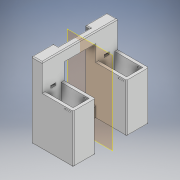
# Autodesk Inventor part: caja_s
Saved by Autodesk Inventor 2020 (Build 240168000, 168)
## iProperties
Created: 2021-01-14
Part Number: caja_s
Material: Generic
Document SubType Name: Modeling
Designer: Gelect
Density: 1 g/cm^3
Appearance: Default
Author: Gelect
Autodesk Inventor part; units mm, degrees
ref_plane "YZ Plane" through (0, 0, 0) normal (1, 0, 0) x (0, 1, 0)
ref_plane "XZ Plane" through (0, 0, 0) normal (0, 1, 0) x (-1, 0, 0)
ref_plane "XY Plane" through (0, 0, 0) normal (0, 0, 1) x (1, 0, 0)
sketch "Sketch1" plane through (0, 0, 0) normal (1, 0, 0) x (0, 1, 0)
  line L0 (38.75, 38.75) -> (-38.75, 38.75)
  line L1 (-38.75, 38.75) -> (-38.75, -38.75)
  line L2 (-38.75, -38.75) -> (38.75, -38.75)
  line L3 (38.75, -38.75) -> (38.75, 38.75)
  line L4 (38.75, 38.75) -> (-38.75, -38.75) construction
  line L5 (-38.75, 38.75) -> (38.75, -38.75) construction
  line L6 (38.75, 16.15) -> (-38.75, 16.15)
  line L7 (-38.75, 16.15) -> (-38.75, -16.15)
  line L8 (-38.75, -16.15) -> (38.75, -16.15)
  line L9 (38.75, -16.15) -> (38.75, 16.15)
  line L10 (38.75, 16.15) -> (-38.75, -16.15) construction
  line L11 (-38.75, 16.15) -> (38.75, -16.15) construction
  line L12 (27, 38.75) -> (-27, 38.75)
  line L13 (-27, 38.75) -> (-27, -38.75)
  line L14 (-27, -38.75) -> (27, -38.75)
  line L15 (27, -38.75) -> (27, 38.75)
  line L16 (27, 38.75) -> (-27, -38.75) construction
  line L17 (-27, 38.75) -> (27, -38.75) construction
  point P0 (0, 0)
  point P1 (27, 16.15)
  point P2 (27, -16.15)
  point P3 (-27, -16.15)
  point P4 (-27, 16.15)
  dimension "d0" = 77.5
  dimension "d1" = 77.5
  dimension "d2" = 32.3
  dimension "d3" = 54
  constraints: 36 end point, 6 midpoint, 6 parallel, 3 horizontal, 3 perpendicular, 2 point on line
  measures "d0" distance of L2.end L0.start
  measures "d1" distance of L1.end L2.end
  measures "d2" distance between parallel lines of L8 L6
  measures "d3" distance between parallel lines of L13 L15
extrude "Extrusion1" add sketch "Sketch1" along normal blind 11 contours L3 L6 L15 L0 | L15 L6 L13 L0 | L3 L8 L15 L6 | L13 L6 L1 L0 | L3 L2 L15 L8 | L13 L8 L1 L6 | L15 L2 L13 L8 | L13 L2 L1 L8
sketch "Sketch2" plane through (11, 0, 0) normal (1, 0, 0) x (0, 0, -1)
  line L0 (-38.75, -38.75) -> (38.75, -38.75) projected
  line L1 (-38.75, 38.75) -> (38.75, 38.75)
  line L2 (38.75, 38.75) -> (38.75, -38.75)
  line L3 (38.75, -38.75) -> (-38.75, -38.75)
  line L4 (-38.75, -38.75) -> (-38.75, 38.75)
  line L5 (-38.75, 38.75) -> (38.75, -38.75) construction
  line L6 (38.75, 38.75) -> (-38.75, -38.75) construction
  line L7 (-16.15, 38.75) -> (16.15, 38.75)
  line L8 (16.15, 38.75) -> (16.15, -38.75)
  line L9 (16.15, -38.75) -> (-16.15, -38.75)
  line L10 (-16.15, -38.75) -> (-16.15, 38.75)
  line L11 (-16.15, 38.75) -> (16.15, -38.75) construction
  line L12 (16.15, 38.75) -> (-16.15, -38.75) construction
  line L13 (38.75, -38.75) -> (38.75, 38.75) projected
  line L14 (38.75, 11.25) -> (-38.75, 11.25)
  line L15 (-38.75, 38.75) -> (-38.75, -38.75) projected
  point P0 (0, 0)
  point P1 (-38.75, -38.75)
  point P2 (-16.15, 11.25)
  point P3 (-38.75, 11.25)
  point P4 (16.15, 11.25)
  dimension "d6" = 32.3
  dimension "d7" = 77.5
  dimension "d25" = 50
  constraints: 26 end point, 4 midpoint, 4 parallel, 3 perpendicular, 3 point on line, 2 horizontal
  measures "d6" distance between parallel lines of L8 L10
  measures "d7" distance of L1.start L1.end
  measures "d25" distance between parallel lines of L0 L14
extrude "Extrusion2" add sketch "Sketch2" along normal blind 31.8 contours L4 L14 L10 L0 | L8 L14 L2 L0
sketch "Sketch5" plane through (0, 38.75, 38.75) normal (0, 1, 0) x (1, 0, 0)
  line L0 (0, 54.9) -> (11, 54.9) projected
  line L1 (-5, 22.6) -> (5, 22.6)
  line L2 (5, 22.6) -> (5, 54.9)
  line L3 (5, 54.9) -> (-5, 54.9)
  line L4 (-5, 54.9) -> (-5, 22.6)
  line L5 (-5, 22.6) -> (5, 54.9) construction
  line L6 (5, 22.6) -> (-5, 54.9) construction
  point P0 (0, 38.75)
  dimension "d16" = 5
  constraints: 12 end point, 2 midpoint, 2 parallel, 1 horizontal, 1 perpendicular, 1 point on line
  measures "d16" distance from line of L2 point (0, 38.75)
extrude "Extrusion4" cut sketch "Sketch5" against normal through all
sketch "Sketch6" plane through (0, 38.75, 38.75) normal (0, 1, 0) x (1, 0, 0)
  line L0 (11, 22.6) -> (42.8, 22.6) projected
  line L1 (0, 0) -> (42.8, 0) projected
  line L2 (42.8, 22.6) -> (11, 22.6)
  line L3 (11, 22.6) -> (11, 0)
  line L4 (11, 0) -> (42.8, 0)
  line L5 (42.8, 0) -> (42.8, 22.6)
  line L6 (11, 22.6) -> (11, 54.9) projected
  line L7 (0, 77.5) -> (42.8, 77.5) projected
  line L8 (11, 54.9) -> (42.8, 54.9)
  line L9 (42.8, 54.9) -> (42.8, 77.5)
  line L10 (42.8, 77.5) -> (11, 77.5)
  line L11 (11, 77.5) -> (11, 54.9)
  line L12 (14, 3) -> (14, 19.6)
  line L13 (14, 19.6) -> (39.8, 19.6)
  line L14 (39.8, 19.6) -> (39.8, 3)
  line L15 (39.8, 3) -> (14, 3)
  line L16 (39.8, 57.9) -> (14, 57.9)
  line L17 (14, 57.9) -> (14, 74.5)
  line L18 (14, 74.5) -> (39.8, 74.5)
  line L19 (39.8, 74.5) -> (39.8, 57.9)
  line L20 (14, 3) -> (11, 3)
  line L21 (14, 19.6) -> (11, 19.6)
  line L22 (14, 57.9) -> (11, 57.9)
  line L23 (11, 54.9) -> (11, 77.5) projected
  line L24 (14, 74.5) -> (11, 74.5)
  point P0 (0, 38.75)
  dimension "d19" = 31.8
  dimension "d20" = 3
  dimension "d21" = 3
  constraints: 40 end point, 9 parallel, 6 perpendicular, 5 point on line, 3 horizontal, 6 other
  measures "d19" distance of L4.end L3.end
  measures "d20" distance between parallel lines of L3 L12
  measures "d21" distance between parallel lines of L8 L16
extrude "Extrusion5" cut sketch "Sketch6" against normal blind 74.5 contours L21 L12 L20 L3 | L13 L14 L15 L12 | L24 L17 L22 L11 | L18 L19 L16 L17
fillet "Fillet1" radius 1 32 edges at (5, 38.75, 0) (0, 38.75, -27.45) (0, 0, -38.75) (5.5, 38.75, -38.75) (2.5, 38.75, -16.15) (11, 38.75, 0) (2.5, 38.75, 16.15) (42.8, -13.75, 16.15) (0, 0, 16.15) (0, 38.75, 27.45) (5, 27, 0) (5.5, 38.75, 38.75) (0, 0, 38.75) (0, 0, -16.15) (5, -27, 0) (11, -27, 0) (5, -38.75, 0) (0, -38.75, 27.45) (2.5, -38.75, 16.15) (26.9, -38.75, 16.15) (0, -38.75, -27.45) (21.4, -38.75, -38.75) (42.8, -13.75, -38.75) (11, 27, 0) (26.9, -38.75, -16.15) (21.4, -38.75, 38.75) (42.8, -13.75, 38.75) (42.8, -38.75, 27.45) (42.8, -13.75, -16.15) (42.8, -38.75, -27.45) (2.5, -38.75, -16.15) (11, -38.75, 0)
sketch "Sketch7" plane through (11, 0, 0) normal (1, 0, 0) x (0, 0, -1)
  line L0 (-17.15, 11.25) -> (-37.75, 11.25) projected
  line L1 (-29.95, 11.25) -> (-24.95, 11.25)
  line L2 (-24.95, 11.25) -> (-24.95, 13.75)
  line L3 (-24.95, 13.75) -> (-29.95, 13.75)
  line L4 (-29.95, 13.75) -> (-29.95, 11.25)
  line L5 (-38.75, 37.75) -> (-38.75, 11.25) projected
  point P0 (0, 0)
  dimension "d26" = 2.5
  dimension "d27" = 5
  dimension "d28" = 8.8
  constraints: 8 end point, 2 parallel, 1 horizontal, 1 perpendicular, 1 point on line
  measures "d26" distance of L1.end L2.end
  measures "d27" distance of L2.end L3.end
  measures "d28" distance between parallel lines of L5 L4
extrude "Extrusion6" cut sketch "Sketch7" against normal through all
ref_plane "Work Plane1" through (1, -37.75, 0) normal (0, 0, 1) x (1, 0, 0)
mirror "Mirror1" about plane through (1, -37.75, 0) normal (0, 0, 1) of "Extrusion6"
sketch "Sketch8" plane through (1, -37.75, 38.75) normal (0, 0, 1) x (1, 0, 0)
  line L0 (33.3, 47.5) -> (38.8, 47.5)
  line L1 (38.8, 47.5) -> (38.8, 46.5)
  line L2 (38.8, 46.5) -> (33.3, 46.5)
  line L3 (33.3, 46.5) -> (33.3, 47.5)
  line L4 (41.8, 0) -> (41.8, 49) projected
  line L5 (10, 49) -> (40.8, 49) projected
  point P0 (-1, 37.75)
  dimension "d31" = 3
  dimension "d32" = 1.5
  dimension "d33" = 1
  dimension "d34" = 5.5
  constraints: 8 end point, 2 parallel, 1 horizontal, 1 perpendicular
  measures "d31" distance between parallel lines of L4 L1
  measures "d32" distance between parallel lines of L5 L0
  measures "d33" distance of L2.end L0.start
  measures "d34" distance of L1.end L2.end
extrude "Extrusion7" cut sketch "Sketch8" against normal through all
equation "\"d1\" = d0"
body "Solid1"
